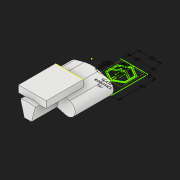
# Autodesk Inventor part: Body
Saved by Autodesk Inventor 2017 SP1 (Build 210196100, 196)
## iProperties
Created: 2018-03-03
Part Number: Body
Material: Generic
Document SubType Name: Modeling
Designer: Zach
Density: 1 g/cm^3
Appearance: CR White
Author: Zach
Autodesk Inventor part; units mm, degrees
ref_plane "YZ Plane" through (0, 0, 0) normal (1, 0, 0) x (0, 1, 0)
ref_plane "XZ Plane" through (0, 0, 0) normal (0, 1, 0) x (-1, 0, 0)
ref_plane "XY Plane" through (0, 0, 0) normal (0, 0, 1) x (1, 0, 0)
sketch "Sketch1" plane through (0, 0, 0) normal (0, 0, 1) x (1, 0, 0)
  line L0 (106.5, -56.5) -> (106.5, 56.5)
  line L1 (38.589, -78.0481) -> (135.1815, -103.93)
  circle A0 centre (155.8871, -26.656) radius 5.25
  line L2 (80, 76.5) -> (176.5926, 50.6181)
  circle A1 centre (155.8871, -26.656) radius 80 construction
  arc A2 (135.1815, -103.93) -> (176.5926, 50.6181) centre (155.8871, -26.656) ccw
  circle A3 centre (-155.8871, -26.656) radius 80 construction
  line L3 (-176.5926, 50.6181) -> (-80, 76.5)
  circle A4 centre (-155.8871, -26.656) radius 5.25
  arc A5 (-176.5926, 50.6181) -> (-135.1815, -103.93) centre (-155.8871, -26.656) ccw
  line L4 (-106.5, 56.5) -> (-106.5, -56.5)
  line L5 (80, 76.5) -> (38.589, -78.0481) construction
  circle A6 centre (0, 71.664) radius 5.25
  line L6 (-38.589, -78.0481) -> (38.589, -78.0481)
  line L7 (-80, 76.5) -> (-38.589, -78.0481) construction
  line L8 (-135.1815, -103.93) -> (-38.589, -78.0481)
  line L9 (-106.5, -56.5) -> (106.5, -56.5)
  line L10 (106.5, 56.5) -> (-106.5, 56.5)
  line L11 (-80, 76.5) -> (80, 76.5) construction
  arc A7 (80, 76.5) -> (-80, 76.5) centre (0, -228.172) ccw
  line L12 (310, 185.5) -> (-310, 185.5) construction
  line L13 (0, 185.5) -> (0, 0) construction
  line L14 (0, 0) -> (310, 0) construction
  line L15 (310, 75.5) -> (310, -324.5) construction
  line L16 (0, -78.0481) -> (0, -56.5)
  point P0 (0, 0)
  point P1 (0, 76.5)
  point P2 (-106.5, 0)
  dimension "d0" = 160
  dimension "d1" = 100
  dimension "d2" = 100
  dimension "d3" = 160
  dimension "d4" = 160
  dimension "d5" = 160
  dimension "d6" = 75
  dimension "d7" = 75
  dimension "d8" = 160
  dimension "d9" = 100
  dimension "d10" = 100
  dimension "d11" = 10.5
  dimension "d12" = 10.5
  dimension "d13" = 113
  dimension "d14" = 213
  dimension "d15" = 20
  dimension "d16" = 315
  dimension "d17" = 10.5
  dimension "d18" = 15.164
  dimension "d19" = 185.5
  constraints: 34 end point, 10 point on circle, 8 centre point, 8 tangent, 5 coincident, 5 midpoint, 3 perpendicular, 2 parallel, 2 point on line, 2 vertical alignment, 1 horizontal alignment, 1 vertical
  measures "d0" diameter of A3
  measures "d1" distance of L11.start L3.start
  measures "d2" distance of L6.start L8.start
  measures "d3" distance of L11.start L6.start
  measures "d4" distance of L11.start L11.end
  measures "d5" distance of L11.end L6.end
  measures "d6" angle of L11 L7
  measures "d7" angle of L11 L5
  measures "d8" diameter of A1
  measures "d9" distance of L6.end L1.end
  measures "d10" distance of L11.end L2.end
  measures "d11" diameter of A4
  measures "d12" diameter of A0
  measures "d13" distance of L10.start L9.end
  measures "d14" distance of L9.end L9.start
  measures "d15" distance between parallel lines of L11 L10
  measures "d16" radius of A7
  measures "d17" diameter of A6
  measures "d18" distance from line of L10 A6.centre
  measures "d19" distance of L13.start L13.end
extrude "Extrusion1" add sketch "Sketch1" along normal blind 415 contours L9 L4 L10 L0 | L6 L8 A5 L3 A7 L2 A2 L1 | A0 | A4 | A6
sketch "Sketch2" plane through (0, 0, 415) normal (0, 0, 1) x (1, 0, 0)
  line L0 (-38.589, -78.0481) -> (38.589, -78.0481) projected
  line L1 (-80, 76.5) -> (-176.5926, 50.6181) projected
  line L2 (-38.589, -78.0481) -> (-80, 76.5)
  line L3 (176.5926, 50.6181) -> (80, 76.5) projected
  line L4 (38.589, -78.0481) -> (80, 76.5)
  arc A0 (80, 76.5) -> (-80, 76.5) centre (0, -228.172) ccw projected
  point P0 (0, 0)
  constraints: 4 end point, 2 perpendicular
extrude "Extrusion2" add sketch "Sketch2" along normal blind 275
ref_plane "Work Plane1" through (-38.589, 76.9519, 0) normal (0, -1, 0) x (1, 0, 0)
sketch "Sketch3" plane through (-38.589, 76.9519, 0) normal (0, -1, 0) x (1, 0, 0)
  line L0 (188.589, 642.5) -> (-111.411, 642.5)
  line L1 (-111.411, 642.5) -> (-111.411, 242.5)
  line L2 (-111.411, 242.5) -> (188.589, 242.5)
  line L3 (188.589, 242.5) -> (188.589, 642.5)
  line L4 (118.589, 690) -> (-41.411, 690) projected
  point P0 (38.589, 0)
  point P1 (38.589, 642.5)
  point P2 (38.589, 690)
  dimension "d25" = 300
  dimension "d26" = 400
  dimension "d27" = 47.5
  constraints: 8 end point, 2 midpoint, 2 parallel, 1 horizontal, 1 perpendicular, 1 vertical alignment
  measures "d25" distance of L2.end L1.end
  measures "d26" distance of L1.end L0.end
  measures "d27" distance between parallel lines of L4 L0
extrude "Extrusion3" add sketch "Sketch3" against normal blind 72
sketch "Sketch4" plane through (-38.589, 148.9519, 0) normal (0, 1, 0) x (1, 0, 0)
  line L0 (188.589, -107.5) -> (488.589, -107.5) construction
  line L1 (488.589, -107.5) -> (488.589, -242.5) construction
  line L2 (488.589, -242.5) -> (188.589, -242.5) construction
  line L3 (188.589, -242.5) -> (188.589, -107.5) construction
  line L4 (213.589, 142.5) -> (463.589, 142.5) construction
  line L5 (463.589, 142.5) -> (463.589, -107.5) construction
  line L6 (463.589, -107.5) -> (213.589, -107.5) construction
  line L7 (213.589, -107.5) -> (213.589, 142.5) construction
  line L8 (488.589, 157.5) -> (188.589, 157.5)
  line L9 (488.589, -242.5) -> (488.589, 157.5)
  line L10 (338.589, 142.5) -> (446.8421, 80)
  line L11 (446.8421, 80) -> (446.8421, -45)
  line L12 (446.8421, -45) -> (338.589, -107.5)
  line L13 (338.589, -107.5) -> (230.3358, -45)
  line L14 (230.3358, -45) -> (230.3358, 80)
  line L15 (230.3358, 80) -> (338.589, 142.5)
  line L16 (338.589, 130.7221) -> (436.6421, 74.111)
  line L17 (436.6421, 74.111) -> (436.6421, -39.111)
  line L18 (436.6421, -39.111) -> (338.589, -95.7221)
  line L19 (338.589, -95.7221) -> (240.5358, -39.111)
  line L20 (240.5358, -39.111) -> (240.5358, 74.111)
  line L21 (240.5358, 74.111) -> (338.589, 130.7221)
  line L22 (338.589, 125.8146) -> (432.3921, 71.6573) construction
  line L23 (432.3921, 71.6573) -> (432.3921, -36.6573) construction
  line L24 (432.3921, -36.6573) -> (338.589, -90.8146) construction
  line L25 (338.589, -90.8146) -> (244.7858, -36.6573) construction
  line L26 (244.7858, -36.6573) -> (244.7858, 71.6573) construction
  line L27 (244.7858, 71.6573) -> (338.589, 125.8146) construction
  line L28 (244.7858, 19.1573) -> (284.7858, 42.2513)
  line L29 (284.7858, 42.2513) -> (284.7858, 70.7513)
  line L30 (284.7858, 70.7513) -> (298.7858, 70.7513)
  line L31 (298.7858, 70.7513) -> (298.7858, 50.3342)
  line L32 (298.7858, 50.3342) -> (338.589, 73.3146)
  line L33 (338.589, 73.3146) -> (432.3921, 19.1573)
  line L34 (432.3921, 19.1573) -> (432.3921, 71.6573)
  line L35 (432.3921, 71.6573) -> (338.589, 125.8146)
  line L36 (338.589, 125.8146) -> (244.7858, 71.6573)
  line L37 (244.7858, 19.1573) -> (244.7858, 71.6573)
  line L38 (244.7858, -36.6573) -> (326.589, -83.8864)
  line L39 (326.589, -83.8864) -> (326.589, -43.8146)
  line L40 (326.589, -43.8146) -> (350.589, -43.8146)
  line L41 (350.589, -43.8146) -> (350.589, -83.8864)
  line L42 (350.589, -83.8864) -> (432.3921, -36.6573)
  line L43 (432.3921, -36.6573) -> (432.3921, 4.1573)
  line L44 (432.3921, 4.1573) -> (338.589, 58.3146)
  line L45 (338.589, 58.3146) -> (244.7858, 4.1573)
  line L46 (244.7858, 4.1573) -> (244.7858, -36.6573)
  line L47 (312.339, 30.1854) -> (364.839, 30.1854) construction
  line L48 (364.839, 30.1854) -> (364.839, -20.8146) construction
  line L49 (364.839, -20.8146) -> (312.339, -20.8146) construction
  line L50 (312.339, -20.8146) -> (312.339, 30.1854) construction
  line L51 (312.339, -20.8146) -> (336.339, -20.8146)
  line L52 (336.339, -20.8146) -> (336.339, 3.1854)
  line L53 (336.339, 3.1854) -> (312.339, 3.1854)
  line L54 (312.339, 3.1854) -> (312.339, -20.8146)
  line L55 (312.339, 30.1854) -> (336.339, 30.1854)
  line L56 (336.339, 30.1854) -> (336.339, 6.1854)
  line L57 (336.339, 6.1854) -> (312.339, 6.1854)
  line L58 (312.339, 6.1854) -> (312.339, 30.1854)
  line L59 (364.839, 30.1854) -> (340.839, 30.1854)
  line L60 (340.839, 30.1854) -> (340.839, 6.1854)
  line L61 (340.839, 6.1854) -> (364.839, 6.1854)
  line L62 (364.839, 6.1854) -> (364.839, 30.1854)
  line L63 (364.839, -20.8146) -> (340.839, -20.8146)
  line L64 (340.839, -20.8146) -> (340.839, 3.1854)
  line L65 (340.839, 3.1854) -> (364.839, 3.1854)
  line L66 (364.839, 3.1854) -> (364.839, -20.8146)
  line L67 (338.589, 157.5) -> (338.589, 142.5)
  line L68 (338.589, 142.5) -> (338.589, -107.5) construction
  line L69 (188.589, -242.5) -> (-111.411, -242.5) projected
  point P0 (38.589, 0)
  point P1 (338.589, 17.5)
  point P2 (338.589, -43.8146)
  point P3 (338.589, 30.1854)
  point P4 (338.589, -20.8146)
  dimension "d30" = 15
  dimension "d31" = 250
  dimension "d32" = 10.2
  dimension "d33" = 4.25
  dimension "d34" = 52.5
  dimension "d35" = 40
  dimension "d36" = 14
  dimension "d37" = 28.5
  dimension "d38" = 15
  dimension "d39" = 24
  dimension "d40" = 47
  dimension "d41" = 23
  dimension "d42" = 51
  dimension "d43" = 52.5
  dimension "d44" = 24
  dimension "d45" = 24
  dimension "d46" = 24
  dimension "d47" = 24
  dimension "d48" = 24
  dimension "d49" = 24
  dimension "d50" = 24
  dimension "d51" = 24
  dimension "d54" = 300
  dimension "d56" = 400
  constraints: 122 end point, 15 parallel, 14 perpendicular, 12 point on line, 7 midpoint, 4 collinear, 2 coincident, 1 horizontal, 1 vertical, 26 other
  measures "d30" distance between parallel lines of L8 L4
  measures "d31" distance of L7.end L5.start
  measures "d32" distance between parallel lines of L15 L21
  measures "d33" distance between parallel lines of L21 L27
  measures "d34" distance of L28.start L37.end
  measures "d35" distance between parallel lines of L26 L29
  measures "d36" distance of L30.start L30.end
  measures "d37" distance of L29.start L30.start
  measures "d38" distance of L33.start L44.end
  measures "d39" distance between parallel lines of L41 L39
  measures "d40" distance from line of L24.end L40
  measures "d41" distance between parallel lines of L40 L49
  measures "d42" distance of L51.start L55.start
  measures "d43" distance of L55.start L62.end
  measures "d44" distance of L53.end L53.start
  measures "d45" distance of L53.start L51.end
  measures "d46" distance of L56.end L57.end
  measures "d47" distance of L55.end L56.end
  measures "d48" distance of L61.end L61.start
  measures "d49" distance of L61.start L60.start
  measures "d50" distance of L64.end L66.start
  measures "d51" distance of L64.start L64.end
  measures "d54" distance of L9.end L8.end
  measures "d56" distance of L9.start L9.end
body "Solid1"
